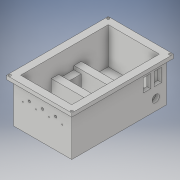
# Autodesk Inventor part: mien_arm
Saved by Autodesk Inventor 2019 (Build 230136000, 136)
## iProperties
Created: 2018-11-23
Part Number: mien_arm
Material: Generic
Document SubType Name: Modeling
Designer: jerem
Density: 1 g/cm^3
Appearance: Default
Author: jerem
Autodesk Inventor part; units mm, degrees
ref_plane "YZ Plane" through (0, 0, 0) normal (1, 0, 0) x (0, 1, 0)
ref_plane "XZ Plane" through (0, 0, 0) normal (0, 1, 0) x (-1, 0, 0)
ref_plane "XY Plane" through (0, 0, 0) normal (0, 0, 1) x (1, 0, 0)
sketch "Sketch1" plane through (0, 0, 0) normal (0, 1, 0) x (-1, 0, 0)
  line L0 (56, 0) -> (-56, 0) projected
  line L1 (0, -156) -> (0, 26) projected
  line L2 (40, 0) -> (-40, 0)
  line L3 (-40, 0) -> (-40, -130)
  line L4 (-40, -130) -> (40, -130)
  line L5 (40, -130) -> (40, 0)
  point P0 (0, 0)
  point P1 (0, 0)
  dimension "d0" = 80
  dimension "d1" = 130
  dimension "d2" = 40
  constraints: 8 end point, 2 midpoint, 2 parallel, 1 horizontal, 1 perpendicular
  measures "d0" distance of L4.end L3.end
  measures "d1" distance of L3.end L2.end
  measures "d2" distance between parallel lines of L5 L1
extrude "Extrusion1" add sketch "Sketch1" along normal blind 60
sketch "Sketch2" plane through (0, 60, 0) normal (0, 1, 0) x (1, 0, 0)
  line L0 (-35, 5) -> (35, 5)
  line L1 (35, 5) -> (35, 125)
  line L2 (35, 125) -> (-35, 125)
  line L3 (-35, 125) -> (-35, 5)
  line L4 (-40, 130) -> (-40, 0) projected
  line L5 (-40, 0) -> (40, 0) projected
  point P0 (0, 0)
  dimension "d5" = 70
  dimension "d6" = 120
  dimension "d7" = 5
  dimension "d8" = 5
  constraints: 8 end point, 2 parallel, 1 horizontal, 1 perpendicular
  measures "d5" distance of L2.end L1.end
  measures "d6" distance of L1.end L0.end
  measures "d7" distance between parallel lines of L4 L3
  measures "d8" distance between parallel lines of L5 L0
extrude "Extrusion2" cut sketch "Sketch2" against normal blind 50
sketch "Sketch3" plane through (40, 0, 0) normal (1, 0, 0) x (0, 0, -1)
  line L0 (113, 48) -> (123, 48)
  line L1 (123, 48) -> (123, 30)
  line L2 (123, 30) -> (113, 30)
  line L3 (113, 30) -> (113, 48)
  line L4 (130, 0) -> (130, 60) projected
  line L5 (0, 60) -> (130, 60) projected
  line L6 (98, 48) -> (108, 48)
  line L7 (108, 48) -> (108, 30)
  line L8 (108, 30) -> (98, 30)
  line L9 (98, 30) -> (98, 48)
  point P0 (0, 0)
  dimension "d11" = 10
  dimension "d12" = 18
  dimension "d13" = 7
  dimension "d14" = 12
  dimension "d15" = 10
  dimension "d16" = 18
  dimension "d17" = 5
  constraints: 16 end point, 4 parallel, 2 horizontal, 2 perpendicular, 1 collinear
  measures "d11" distance of L1.end L2.end
  measures "d12" distance of L0.end L1.end
  measures "d13" distance between parallel lines of L4 L1
  measures "d14" distance between parallel lines of L5 L0
  measures "d15" distance of L7.end L8.end
  measures "d16" distance of L6.end L7.end
  measures "d17" distance between parallel lines of L3 L7
extrude "Extrusion3" cut sketch "Sketch3" against normal blind 5
sketch "Sketch4" plane through (40, 0, 0) normal (1, 0, 0) x (0, 0, -1)
  circle A0 centre (115, 15) radius 5
  line L0 (0, 0) -> (130, 0) projected
  line L1 (130, 0) -> (130, 60) projected
  dimension "d20" = 10
  dimension "d21" = 15
  dimension "d22" = 15
  constraints: 1 centre point
  measures "d20" diameter of A0
  measures "d21" distance from line of A0.centre L0
  measures "d22" distance from line of L1 A0.centre
extrude "Extrusion4" cut sketch "Sketch4" against normal blind 5
sketch "Sketch6" plane through (0, 10, 0) normal (0, 1, 0) x (1, 0, 0)
  line L0 (-35, 125) -> (35, 125) projected
  line L1 (-35, 5) -> (-35, 125) projected
  line L2 (35, 5) -> (-35, 5) projected
  line L3 (35, 115) -> (35, 5) projected
  line L4 (35, 125) -> (35, 115) projected
  line L5 (-35, 88) -> (30, 88)
  line L6 (30, 88) -> (30, 78)
  line L7 (30, 78) -> (-35, 78)
  line L8 (-35, 78) -> (-35, 88)
  line L9 (25, 125) -> (25, 88) projected
  line L10 (25, 88) -> (30, 88) projected
  line L11 (30, 88) -> (30, 125) projected
  point P0 (0, 0)
  dimension "d30" = 65
  dimension "d31" = 10
  constraints: 8 end point, 2 collinear, 2 parallel, 1 horizontal, 1 perpendicular
  measures "d30" distance of L6.end L7.end
  measures "d31" distance of L5.end L6.end
extrude "Extrusion6" add sketch "Sketch6" along normal blind 25 contours L5 L6 L7 L1
sketch "Sketch7" plane through (0, 10, 0) normal (0, 1, 0) x (1, 0, 0)
  line L0 (30, 78) -> (-35, 78) projected
  line L1 (-35, 5) -> (-35, 78) projected
  line L2 (35, 5) -> (-35, 5) projected
  line L3 (35, 115) -> (35, 5) projected
  line L4 (35, 125) -> (35, 115) projected
  line L5 (-35, 125) -> (35, 125) projected
  line L6 (30, 88) -> (30, 78) projected
  line L7 (-35, 57) -> (30, 57)
  line L8 (30, 57) -> (30, 47)
  line L9 (30, 47) -> (-35, 47)
  line L10 (-35, 47) -> (-35, 57)
  line L11 (30, 88) -> (30, 125) projected
  line L12 (-35, 88) -> (30, 88) projected
  line L13 (-35, 88) -> (-35, 125) projected
  point P0 (0, 0)
  dimension "d34" = 65
  dimension "d35" = 10
  dimension "d36" = 21
  constraints: 8 end point, 2 parallel, 1 collinear, 1 horizontal, 1 perpendicular
  measures "d34" distance of L8.end L9.end
  measures "d35" distance of L7.end L8.end
  measures "d36" distance between parallel lines of L7 L0
extrude "Extrusion7" add sketch "Sketch7" along normal blind 25 contours L7 L8 L9 L1
sketch "Sketch8" plane through (0, 10, 0) normal (0, 1, 0) x (1, 0, 0)
  line L0 (-35, 57) -> (30, 57) projected
  line L1 (30, 57) -> (30, 47) projected
  line L2 (30, 47) -> (-35, 47) projected
  line L3 (-35, 5) -> (-35, 47) projected
  line L4 (35, 5) -> (-35, 5) projected
  line L5 (35, 115) -> (35, 5) projected
  line L6 (35, 125) -> (35, 115) projected
  line L7 (-35, 125) -> (35, 125) projected
  line L8 (30, 88) -> (30, 78) projected
  line L9 (30, 78) -> (-35, 78) projected
  line L10 (-35, 57) -> (-35, 78) projected
  line L11 (-35, 78) -> (-25, 78)
  line L12 (-25, 78) -> (-25, 57)
  line L13 (-25, 57) -> (-35, 57)
  line L14 (-35, 57) -> (-35, 78)
  line L15 (16, 58) -> (16, 79)
  line L16 (16, 79) -> (26, 79)
  line L17 (26, 79) -> (26, 57)
  line L18 (26, 57) -> (16, 57)
  line L19 (16, 57) -> (16, 79)
  line L20 (30, 57) -> (-35, 57) projected
  line L21 (-35, 88) -> (-35, 125) projected
  line L22 (-35, 88) -> (30, 88) projected
  point P0 (0, 0)
  dimension "d39" = 10
  dimension "d40" = 10
  dimension "d41" = 41
  constraints: 18 end point, 4 parallel, 2 horizontal, 2 perpendicular, 1 collinear, 1 point on line
  measures "d39" distance between parallel lines of L10 L12
  measures "d40" distance between parallel lines of L15 L17
  measures "d41" distance between parallel lines of L12 L15
extrude "Extrusion8" add sketch "Sketch8" along normal blind 20 contours L10 L9 L12 L0 | L19 L15 L9 L17 L0 | L15 L16 L17 L9
sketch "Sketch10" plane through (-40, 0, 0) normal (0, 0, 1) x (1, 0, 0)
  circle A0 centre (22, 40) radius 1.625
  circle A1 centre (40, 40) radius 1.625
  circle A2 centre (58, 40) radius 1.625
  line L0 (0, 0) -> (0, 60) projected
  line L1 (0, 0) -> (80, 0) projected
  line L2 (80, 0) -> (80, 60) projected
  line L3 (0, 60) -> (80, 60) projected
  line L4 (0, 0) -> (0, 60) projected
  point P0 (40, 0)
  dimension "d49" = 3.25
  dimension "d51" = 3.25
  dimension "d53" = 3.25
  dimension "d55" = 18
  dimension "d56" = 18
  dimension "d59" = 22
  dimension "d60" = 22
  dimension "d61" = 20
  constraints: 3 centre point
  measures "d49" diameter of A0
  measures "d51" diameter of A1
  measures "d53" diameter of A2
  measures "d55" distance of A1.centre A0.centre
  measures "d56" distance of A2.centre A1.centre
  measures "d59" distance from line of L0 A0.centre
  measures "d60" distance from line of L2 A2.centre
  measures "d61" distance from line of L3 A1.centre
extrude "Extrusion10" cut sketch "Sketch10" against normal blind 10 contours A0 | A1 | A2
sketch "Sketch11" plane through (-40, 0, 0) normal (0, 0, 1) x (1, 0, 0)
  circle A0 centre (13, 35) radius 0.75
  circle A1 centre (31, 35) radius 0.75
  circle A2 centre (49, 35) radius 0.75
  circle A3 centre (67, 35) radius 0.75
  circle A4 centre (40, 40) radius 1.625 projected
  circle A5 centre (22, 40) radius 1.625 projected
  circle A6 centre (58, 40) radius 1.625 projected
  line L0 (0, 0) -> (80, 0) projected
  line L1 (80, 0) -> (80, 60) projected
  line L2 (0, 60) -> (80, 60) projected
  line L3 (0, 0) -> (0, 60) projected
  dimension "d64" = 1.5
  dimension "d65" = 1.5
  dimension "d66" = 1.5
  dimension "d67" = 1.5
  dimension "d71" = 18
  dimension "d73" = 18
  dimension "d75" = 18
  dimension "d76" = 13
  dimension "d77" = 13
  dimension "d78" = 5
  dimension "d79" = 5
  constraints: 4 centre point
  measures "d64" diameter of A0
  measures "d65" diameter of A1
  measures "d66" diameter of A2
  measures "d67" diameter of A3
  measures "d71" distance of A0.centre A1.centre
  measures "d73" distance of A2.centre A1.centre
  measures "d75" distance of A3.centre A2.centre
  measures "d76" distance from line of L3 A0.centre
  measures "d77" distance from line of L1 A3.centre
  measures "d78" vertical distance of A1.centre A5.centre
  measures "d79" vertical distance of A4.centre A2.centre
extrude "Extrusion11" cut sketch "Sketch11" against normal blind 10 contours A0 | A1 | A2 | A3
sketch "Sketch12" plane through (0, 60, 0) normal (0, 1, 0) x (1, 0, 0)
  line L0 (-44.75, 134.75) -> (44.75, 134.75)
  line L1 (44.75, 134.75) -> (44.75, -4.75)
  line L2 (44.75, -4.75) -> (-44.75, -4.75)
  line L3 (-44.75, -4.75) -> (-44.75, 134.75)
  line L4 (35, 125) -> (35, 5) projected
  line L5 (35, 5) -> (-35, 5) projected
  line L6 (-35, 5) -> (-35, 125) projected
  line L7 (-35, 125) -> (35, 125) projected
  line L8 (-40, 0) -> (40, 0) projected
  line L9 (40, 0) -> (40, 130) projected
  line L10 (40, 130) -> (-40, 130) projected
  line L11 (-40, 130) -> (-40, 0) projected
  line L12 (-40, 130) -> (-40, 0) projected
  line L13 (-40, 130) -> (40, 130)
  line L14 (40, 130) -> (40, 0)
  line L15 (40, 0) -> (-40, 0)
  line L16 (-40, 0) -> (-40, 130)
  point P0 (0, 0)
  dimension "d82" = 4.75
  dimension "d83" = 4.75
  dimension "d84" = 4.75
  dimension "d85" = 4.75
  constraints: 16 end point, 4 parallel, 2 horizontal, 2 perpendicular
  measures "d82" distance between parallel lines of L0 L10
  measures "d83" distance between parallel lines of L8 L2
  measures "d84" distance between parallel lines of L3 L11
  measures "d85" distance between parallel lines of L1 L9
extrude "Extrusion12" add sketch "Sketch12" against normal blind 5 contours L0 L1 L2 L3
sketch "Sketch15" plane through (0, 55, 0) normal (0, -1, 0) x (1, 0, 0)
  line L0 (40, 0) -> (-40, 0) projected
  line L1 (40, -130) -> (40, 0) projected
  line L2 (-40, -130) -> (40, -130) projected
  line L3 (-40, 0) -> (-40, -130) projected
  line L4 (-44.75, -134.75) -> (44.75, -134.75) projected
  line L5 (44.75, -134.75) -> (44.75, 4.75) projected
  line L6 (44.75, 4.75) -> (-44.75, 4.75) projected
  line L7 (-44.75, 4.75) -> (-44.75, -134.75) projected
  line L8 (-40, 0) -> (40, 0) projected
  line L9 (-40, -130) -> (-40, 0) projected
  line L10 (40, -130) -> (-40, -130) projected
  line L11 (40, 0) -> (40, -130) projected
  circle A0 centre (-42.375, 2.375) radius 1.625
  circle A1 centre (42.375, 2.375) radius 1.625
  circle A2 centre (42.375, -132.375) radius 1.625
  circle A3 centre (-42.375, -132.375) radius 1.625
  point P0 (0, 0)
  dimension "d91" = 3.25
  dimension "d92" = 2.375
  dimension "d93" = 2.375
  dimension "d94" = 3.25
  dimension "d95" = 2.375
  dimension "d96" = 2.375
  dimension "d97" = 3.25
  dimension "d98" = 2.375
  dimension "d99" = 2.375
  dimension "d100" = 3.25
  dimension "d101" = 2.375
  dimension "d102" = 2.375
  constraints: 4 centre point
  measures "d91" diameter of A0
  measures "d92" distance from line of L7 A0.centre
  measures "d93" distance from line of L6 A0.centre
  measures "d94" diameter of A1
  measures "d95" distance from line of L6 A1.centre
  measures "d96" distance from line of L5 A1.centre
  measures "d97" diameter of A2
  measures "d98" distance from line of L4 A2.centre
  measures "d99" distance from line of L5 A2.centre
  measures "d100" diameter of A3
  measures "d101" distance from line of L4 A3.centre
  measures "d102" distance from line of L7 A3.centre
extrude "Extrusion13" cut sketch "Sketch15" against normal blind 5 contours A0 | A1 | A2 | A3
sketch "Sketch16" plane through (0, 30, 0) normal (0, 1, 0) x (1, 0, 0)
  line L0 (16, 78) -> (26, 78) projected
  line L1 (16, 78) -> (16, 57) projected
  line L2 (26, 57) -> (16, 57) projected
  line L3 (26, 57) -> (26, 78) projected
  line L4 (16, 57) -> (16, 78) projected
  line L5 (26, 78) -> (26, 57) projected
  line L6 (16, 74.5) -> (26, 74.5)
  line L7 (26, 74.5) -> (26, 60.5)
  line L8 (26, 60.5) -> (16, 60.5)
  line L9 (16, 60.5) -> (16, 74.5)
  point P0 (0, 0)
  dimension "d105" = 3.5
  dimension "d106" = 3.5
  constraints: 8 end point, 2 parallel, 2 point on line, 1 horizontal, 1 perpendicular
  measures "d105" distance between parallel lines of L0 L6
  measures "d106" distance between parallel lines of L8 L2
extrude "Extrusion14" cut sketch "Sketch16" against normal blind 20 contours L6 L3 L8 L1
body "Solid1"
